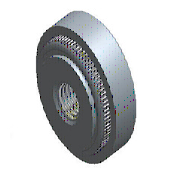
# Autodesk Inventor part: S-M3-0 ZI
Saved by Autodesk Inventor 2019.4 (Build 234330000, 330)
## iProperties
Created: 2018-01-05
Part Number: S-M3-0 ZI
Material: Stal, węglowa
Catalog Web Link: www.pemnet.com
Description: PEM Nakrętki samozaciskowe S,SS,CLS,CLSS - Metryczny
Vendor: PennEngineering®
Document SubType Name: Modeling
Standard: PEM
Designer: barto
Manufacturer: PennEngineering®
Language: pl-PL
Size Designation: S-M3-0 ZI
Categories: <MemberInstance><Categories><Category DisplayName="Blacha" InternalName="21944ee9-ad4d-44c9-9b1e-873eb7935d2a" Mnemonic="PEM"><Category DisplayName="Nakrętki" InternalName="15e34f97-5541-421a-a775-44d98c1adcde" Mnemonic="pemNut"><CategoryParameter DisplayName="Średnica nominalna" InternalName="0be71e27-5492-4f5f-b057-e8c8d33d0305" Mnemonic="nomdia"/><CategoryParameter DisplayName="Klasa gwintu" InternalName="2354338d-f827-46bd-8778-0ed3d7286146" Mnemonic="thrclss"/><CategoryParameter DisplayName="Oznaczenie serii gwintów" InternalName="571a622b-fa51-4821-aeeb-e24f544f017e" Mnemonic="thrserdsgn"/><CategoryParameter DisplayName="Średnica otworu" InternalName="5cda2139-ecc7-4f59-8502-3162f0124b70" Mnemonic="SMNHD"/><CategoryParameter DisplayName="Gwintów na jednostkę" InternalName="64655984-9347-4d07-8751-37792c28ecd8" Mnemonic="thrperunit1"/><CategoryParameter DisplayName="Typ gwintu" InternalName="7a3892cf-1811-453a-b9c2-22c8b70c36bf" Mnemonic="thrtype"/><CategoryParameter DisplayName="Długość gwintu" InternalName="a5235de7-e741-4b6b-b2e9-a6829ffd9d3f" Mnemonic="thrlen"/><CategoryParameter DisplayName="Oznaczenie gwintu" InternalName="ab33a7e4-2ca9-400b-8e2d-5973b7f77f2c" Mnemonic="thrdesign"/><CategoryParameter DisplayName="Głębokość" InternalName="c013d27b-95cd-4187-8e83-a1be557daece" Mnemonic="nheig"/><CategoryParameter DisplayName="Minimalna grubość blachy" InternalName="ff2eaae3-31bc-42d2-bfe3-2e39a04c80e9" Mnemonic="SMNMIST"/></Category></Category><Category DisplayName="TypDanych" InternalName="23b78d0f-2648-40c6-8793-ca6db495c9e8" Mnemonic="DATATYPE"><CategoryParameter DisplayName="NazwaWyświetlana" InternalName="05415f3d-3907-474b-a020-eb9d644f4cf3" Mnemonic="DISPLAYNAME"/><CategoryParameter DisplayName="Standardowe" InternalName="0c0a119c-1e12-4c84-803f-101930972f5e" Mnemonic="STANDARD"/><CategoryParameter DisplayName="Opis" InternalName="13903e3d-64b1-4950-80da-f627842ea37f" Mnemonic="DESCRIPTION"/><CategoryParameter DisplayName="Oznaczenie" InternalName="2675968c-4ce5-49e0-a4f5-552d29089031" Mnemonic="DESIGNATION"/><CategoryParameter DisplayName="Wiersz domyślny" InternalName="2af9ec52-faaa-4026-b378-f9fa4afca842" Mnemonic="DEFAULTROW"/><CategoryParameter DisplayName="Nazwa folderu" InternalName="3f06958e-8713-4116-9be7-ed6184ecc97b" Mnemonic="FOLDERNAME"/><CategoryParameter DisplayName="Wskazówki do poprawek" InternalName="45a75005-10b1-4dfc-8d6d-dfe629f0b93c" Mnemonic="REVISIONGUID"/><CategoryParameter DisplayName="Nazwa pliku" InternalName="8b46a4cc-9585-4fed-90c3-899f57e09a73" Mnemonic="FILENAME"/><CategoryParameter DisplayName="OrgStd" InternalName="8f5914e1-4693-403f-8ab5-d37768198c9d" Mnemonic="STDSORG"/><CategoryParameter DisplayName="Wersja rodziny" InternalName="914462f6-6e19-4b14-ba84-155b9680b1d0" Mnemonic="FAMILYREVISION"/><CategoryParameter DisplayName="Poprawka standardowa" InternalName="91d5a463-65c2-4fde-b823-3b7fea5e8e17" Mnemonic="STANDARDREVISION"/><CategoryParameter DisplayName="Zmiana elementu" InternalName="a65d44b9-392f-4f4f-857b-e4b3d54996fe" Mnemonic="MEMBERREVISION"/><CategoryParameter DisplayName="FormatKlipu" InternalName="bc51e27b-3422-4e78-93ef-cec197ddf230" Mnemonic="CLIPFORMAT"/><CategoryParameter DisplayName="Producent" InternalName="cd6c7a72-a28a-4e50-99a9-2c7f4e13e5ad" Mnemonic="MANUFACTURER"/><CategoryParameter DisplayName="NazwaWewnętrzna" InternalName="cf1d0246-76d9-4b4a-8305-fa0409afb5c1" Mnemonic="INTERNALNAME"/><CategoryParameter DisplayName="CzyMetryczne" InternalName="e2385c5b-1ea4-4823-96a8-8de651266ec3" Mnemonic="ISMETRIC"/><Category DisplayName="Część" InternalName="c0e0b642-3bcb-4cc8-9e80-f96d35c4afa4" Mnemonic="PART"><CategoryParameter DisplayName="Numer części" InternalName="016b6077-bfbe-49bd-92c9-d8d59c39c941" Mnemonic="PARTNUMBER"/><CategoryParameter DisplayName="Numer katalogowy" InternalName="4dba7c1c-e26c-444e-836c-b08b433409a8" Mnemonic="STOCKNUMBER"/><CategoryParameter DisplayName="Klucz - materiał" InternalName="5c9a8adb-dd2b-4535-b97f-0a94a95fe41f" Mnemonic="MATERIALKEY"/><CategoryParameter DisplayName="Materiał" InternalName="818a152a-d3c3-49ca-80ee-df7d91421b8e" Mnemonic="MATERIAL"/></Category></Category></Categories><FamilyTemplate Id="PEM Self-Clinching Nuts S,SS,CLS,CLSS - Metric"><FamilyTemplateParameters><FamilyTemplateParameter ObjectType="kUserParameterObject" ValueType="xs:double" Id="1" ObjectReferenceKey="A_"/><FamilyTemplateParameter ObjectType="kUserParameterObject" ValueType="xs:double" Id="2" ObjectReferenceKey="C1"/><FamilyTemplateParameter ObjectType="kUserParameterObject" ValueType="xs:double" Id="3" ObjectReferenceKey="C_"/><FamilyTemplateParameter ObjectType="kUserParameterObject" ValueType="xs:double" Id="4" ObjectReferenceKey="E_"/><FamilyTemplateParameter ObjectType="kUserParameterObject" ValueType="xs:double" Id="5" ObjectReferenceKey="Height"/><FamilyTemplateParameter ObjectType="kUserParameterObject" ValueType="xs:double" Id="10" ObjectReferenceKey="H_Size"/><FamilyTemplateParameter ObjectType="kUserParameterObject" ValueType="xs:double" Id="11" ObjectReferenceKey="K_"/><FamilyTemplateParameter ObjectType="kUserParameterObject" ValueType="xs:double" Id="13" ObjectReferenceKey="Min_Dist"/><FamilyTemplateParameter ObjectType="kUserParameterObject" ValueType="xs:double" Id="14" ObjectReferenceKey="Min_Thick"/><FamilyTemplateParameter ObjectType="kUserParameterObject" ValueType="xs:double" Id="15" ObjectReferenceKey="NND"/><FamilyTemplateParameter ObjectType="kUserParameterObject" ValueType="xs:double" Id="17" ObjectReferenceKey="T_"/><FamilyTemplateParameter ObjectType="kPropertyObject" ValueType="xs:string" Id="100" ObjectReferenceKey="{32853F0F-3444-11d1-9E93-0060B03C1CA6}" SubObjectId="52"/><FamilyTemplateParameter ObjectType="kPropertyObject" ValueType="xs:string" Id="105" ObjectReferenceKey="{32853F0F-3444-11d1-9E93-0060B03C1CA6}" SubObjectId="5"/><FamilyTemplateParameter ObjectType="kPartComponentDefinitionObject" ValueType="xs:string" Id="110" SubObjectId="Material"/><FamilyTemplateParameter ObjectType="kThreadFeatureObject" ValueType="xs:structure" Id="300" ObjectReferenceKey="1002000010000000da070000000000008000000000000000" SubObjectId="ThreadInfo"><FamilyTemplateParameter ObjectType="" ValueType="xs:string" Id="301" SubObjectId="ThreadClass"/><FamilyTemplateParameter ObjectType="" ValueType="xs:string" Id="302" SubObjectId="ThreadDesignation"/><FamilyTemplateParameter ObjectType="" ValueType="xs:string" Id="303" SubObjectId="ThreadType"/><FamilyTemplateParameter ObjectType="" ValueType="xs:string" Id="304" SubObjectId="Pitch"/><FamilyTemplateParameter ObjectType="" ValueType="xs:string" Id="305" SubObjectId="ThreadType"/></FamilyTemplateParameter></FamilyTemplateParameters></FamilyTemplate><CategoryParameterMap><ParamToTemplateMap><ParamToTemplate CategoryParameter="//CategoryParameter[@InternalName='05415f3d-3907-474b-a020-eb9d644f4cf3']" ConstantValue="PEM Self-Clinching Nuts S,SS,CLS,CLSS - Metric"/><ParamToTemplate CategoryParameter="//CategoryParameter[@InternalName='0c0a119c-1e12-4c84-803f-101930972f5e']" ConstantValue="PEM"/><ParamToTemplate CategoryParameter="//CategoryParameter[@InternalName='13903e3d-64b1-4950-80da-f627842ea37f']" ConstantValue="PEM Self-Clinching Nuts S,SS,CLS,CLSS - Metric"/><ParamToTemplate CategoryParameter="//CategoryParameter[@InternalName='2af9ec52-faaa-4026-b378-f9fa4afca842']" ConstantValue="1"/><ParamToTemplate CategoryParameter="//CategoryParameter[@InternalName='3f06958e-8713-4116-9be7-ed6184ecc97b']" ConstantValue="PEM Self-Clinching Nuts S,SS,CLS,CLSS - Metric"/><ParamToTemplate CategoryParameter="//CategoryParameter[@InternalName='45a75005-10b1-4dfc-8d6d-dfe629f0b93c']" ConstantValue="9c150bdb-5582-4df9-95cc-657864c11748"/><ParamToTemplate CategoryParameter="//CategoryParameter[@InternalName='8f5914e1-4693-403f-8ab5-d37768198c9d']" TemplateParameter="101"/><ParamToTemplate CategoryParameter="//CategoryParameter[@InternalName='914462f6-6e19-4b14-ba84-155b9680b1d0']" ConstantValue="11"/><ParamToTemplate CategoryParameter="//CategoryParameter[@InternalName='91d5a463-65c2-4fde-b823-3b7fea5e8e17']" TemplateParameter="103"/><ParamToTemplate CategoryParameter="//CategoryParameter[@InternalName='bc51e27b-3422-4e78-93ef-cec197ddf230']" ConstantValue="CF_INVENTOR.STDPARTS"/><ParamToTemplate CategoryParameter="//CategoryParameter[@InternalName='cd6c7a72-a28a-4e50-99a9-2c7f4e13e5ad']" ConstantValue="PennEngineering®"/><ParamToTemplate CategoryParameter="//CategoryParameter[@InternalName='cf1d0246-76d9-4b4a-8305-fa0409afb5c1']" ConstantValue="e52ab5ca-f3e0-4e02-85b9-e19727fb1cfc"/><ParamToTemplate CategoryParameter="//CategoryParameter[@InternalName='e2385c5b-1ea4-4823-96a8-8de651266ec3']" ConstantValue="true"/><ParamToTemplate CategoryParameter="//CategoryParameter[@InternalName='7a3892cf-1811-453a-b9c2-22c8b70c36bf']" ConstantValue=""/><ParamToTemplate CategoryParameter="//CategoryParameter[@InternalName='8b46a4cc-9585-4fed-90c3-899f57e09a73']" ConstantValue="S-M3-0 ZI"/><ParamToTemplate CategoryParameter="//CategoryParameter[@InternalName='a65d44b9-392f-4f4f-857b-e4b3d54996fe']" ConstantValue="7e720b2c-8961-4824-87d8-edf765878924"/><ParamToTemplate CategoryParameter="//CategoryParameter[@InternalName='2675968c-4ce5-49e0-a4f5-552d29089031']" TemplateParameter="100"/><ParamToTemplate CategoryParameter="//CategoryParameter[@InternalName='5cda2139-ecc7-4f59-8502-3162f0124b70']" TemplateParameter="10"/><ParamToTemplate CategoryParameter="//CategoryParameter[@InternalName='a5235de7-e741-4b6b-b2e9-a6829ffd9d3f']" TemplateParameter="5"/><ParamToTemplate CategoryParameter="//CategoryParameter[@InternalName='c013d27b-95cd-4187-8e83-a1be557daece']" TemplateParameter="5"/><ParamToTemplate CategoryParameter="//CategoryParameter[@InternalName='2354338d-f827-46bd-8778-0ed3d7286146']" TemplateParameter="301"/><ParamToTemplate CategoryParameter="//CategoryParameter[@InternalName='ab33a7e4-2ca9-400b-8e2d-5973b7f77f2c']" TemplateParameter="302"/><ParamToTemplate CategoryParameter="//CategoryParameter[@InternalName='818a152a-d3c3-49ca-80ee-df7d91421b8e']" TemplateParameter="110"/><ParamToTemplate CategoryParameter="//CategoryParameter[@InternalName='ff2eaae3-31bc-42d2-bfe3-2e39a04c80e9']" TemplateParameter="14"/><ParamToTemplate CategoryParameter="//CategoryParameter[@InternalName='0be71e27-5492-4f5f-b057-e8c8d33d0305']" TemplateParameter="15"/><ParamToTemplate CategoryParameter="//CategoryParameter[@InternalName='016b6077-bfbe-49bd-92c9-d8d59c39c941']" TemplateParameter="105"/></ParamToTemplateMap></CategoryParameterMap></MemberInstance>
Density: 7.85 g/cm^3
Appearance: Częściowo polerowana
IsCustomPart: 0
Title: Nut
Author: barto
Autodesk Inventor part; units mm, degrees
ref_plane "YZ Plane" through (0, 0, 0) normal (1, 0, 0) x (0, 1, 0)
ref_plane "XZ Plane" through (0, 0, 0) normal (0, 1, 0) x (-1, 0, 0)
ref_plane "XY Plane" through (0, 0, 0) normal (0, 0, 1) x (1, 0, 0)
sketch "Sketch2" plane through (0, 0, 0) normal (0, 1, 0) x (-1, 0, 0)
  line L0 (0, 0) -> (0, 2.27)
  line L1 (0, 0) -> (3.15, 0)
  line L2 (3.15, 0) -> (3.15, 1.5)
  line L3 (3.15, 1.5) -> (2.73, 1.5)
  line L4 (2.73, 1.5) -> (2.73, 1.885)
  line L5 (2.73, 1.885) -> (2.4607, 1.885)
  line L6 (2.11, 2.0775) -> (2.11, 2.27)
  line L7 (2.11, 2.27) -> (0, 2.27)
  line L8 (2.11, 2.0775) -> (1.9411, 1.785)
  line L9 (1.9411, 1.785) -> (2.403, 1.785)
  line L10 (2.403, 1.785) -> (2.4607, 1.885)
  dimension "d0" = 1.5
  dimension "d1" = 0.77
  dimension "d2" = 4.22
  dimension "d3" = 6.3
  dimension "d17" = 0.385
  dimension "d18" = 5.46
  dimension "d19" = 0.1925
  dimension "d20" = 30
  dimension "d21" = 0.1
  dimension "d23" = 0.4
  constraints: 22 end point, 5 parallel, 3 perpendicular, 1 vertical
  measures "d0" distance between parallel lines of L3 L1
  measures "d1" distance between parallel lines of L7 L3
  measures "d2" diameter of L6 L0
  measures "d3" diameter of L2 L0
  measures "d17" distance between parallel lines of L5 L3
  measures "d18" diameter of L4 L0
  measures "d19" distance from line of L6.start L7
  measures "d20" angle of L8 L6
  measures "d21" distance between parallel lines of L5 L9
  measures "d23" distance between parallel lines of L10 L8
revolve "Obrót1" add sketch "Sketch2" angle 360 about axis through (0, 0, 0) along (0, 0, 1)
hole "Otwór1" at (0, 0, 2.27) direction (0, 0, -1) diameter 2.459 end through all thread size "M3x0.5" class "6H" standard "ANSI Metric M Profile"
chamfer "Faza1" distance 0.2 angle 45 3 edges at (0, 1.2295, 0) (3.15, 0, 0) (0, 1.2295, 2.27)
equation "\"d14\" = C1"
equation "\"d0\" = T_"
equation "\"d1\" = A_"
equation "\"d2\" = C_"
equation "\"d3\" = E_"
equation "\"d17\" = 0.5 * A_"
equation "\"d19\" = 0.25 * A_"
equation "\"A_\" = 0.77"
equation "\"C_\" = 4.22"
equation "\"E_\" = 6.3"
equation "\"T_\" = 1.5"
equation "\"K_\" = 0.2"
equation "\"C1\" = 0.2"
equation "\"Min_Dist\" = 4.8"
equation "\"H_Size\" = 4.25"
equation "\"Min_Thick\" = 0.8"
equation "\"NND\" = 3"
equation "\"Height\" = 2.27"
body "Solid1"
